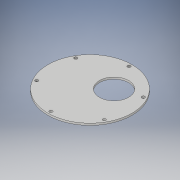
# Autodesk Inventor part: Dremel_Jig_External
Saved by Autodesk Inventor 2018 (Build 220112000, 112)
## iProperties
Created: 2020-08-31
Part Number: Dremel_Jig_External
Material: Generic
Document SubType Name: Modeling
Designer: Ian
Density: 1 g/cm^3
Appearance: Default
Author: Ian
Autodesk Inventor part; units mm, degrees
ref_plane "YZ Plane" through (0, 0, 0) normal (1, 0, 0) x (0, 1, 0)
ref_plane "XZ Plane" through (0, 0, 0) normal (0, 1, 0) x (-1, 0, 0)
ref_plane "XY Plane" through (0, 0, 0) normal (0, 0, 1) x (1, 0, 0)
sketch "Sketch1" plane through (0, 0, 0) normal (0, 1, 0) x (-1, 0, 0)
  circle A0 centre (0, 0) radius 44.45
  circle A1 centre (0, -41.275) radius 1.6
  circle A2 centre (35.7452, -20.6375) radius 1.6
  circle A3 centre (-35.7452, -20.6375) radius 1.6
  circle A4 centre (0, 41.275) radius 1.6
  circle A5 centre (35.7452, 20.6375) radius 1.6
  circle A6 centre (-35.7452, 20.6375) radius 1.6
  circle A7 centre (-12.7279, -12.7279) radius 15.4558
  constraints: 8 centre point
extrude "Extrusion2" add sketch "Sketch1" along normal blind 2
body "Solid2"
